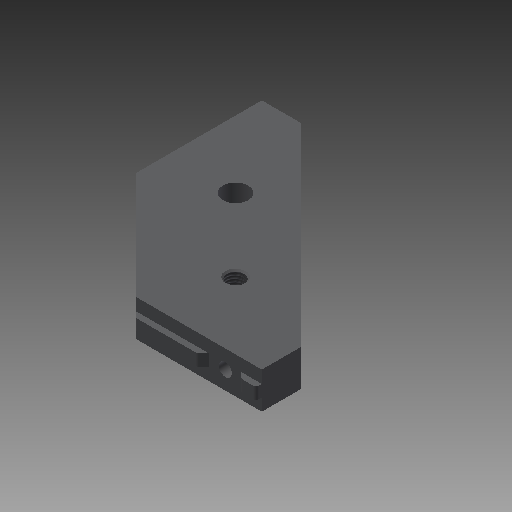
# Autodesk Inventor part: May Tec 1.47.225160.2_Floor mounting plate_schwarz-Pulverbeschichtet
Saved by Autodesk Inventor 2018 (Build 220112000, 112)
## iProperties
Category: PARTsolutions
Company: MAYTEC
Created: 2012-12-06
Part Number: May Tec 1.47.225160.2_Floor mounting plate_schwarz-Pulverbeschichtet
Catalog Web Link: www.cadenas.de
Description: Floor mounting plate-Floor mounting plate
Vendor: MAYTEC
Document SubType Name: Modeling
Designer: PARTuser1
Manufacturer: MAYTEC
Density: 1 g/cm^3
Material: Generic
Appearance: RGB(30.59999931603645,30.59999931603645,30.59999931603645)
PSOL_IDENT_0: {\\10.0.0.242\data_v9\23d-libs\maytec\maytec_3d\einbauzubehoer\platten\1.47.225.prj},292 {VTYP=3D},{
PSOL_IDENT_1: NB=May Tec 1.47.225160.2_Floor mounting plate_schwarz-Pulverbeschichtet},{LINA=May Tec 1.47.225160.2
PSOL_IDENT_2: _Floor mounting plate_schwarz-Pulverbeschichtet},{NN=Floor mounting plate},{DATE=14.09.2010 08:34:44
PSOL_IDENT_3: },{GEOMDATE=28.01.2010 00:00:00},{VERSION=},{LINEID=20},{LINESUBID=-1},{WBVAR=}  {NB=May Tec 1.47.22
PSOL_IDENT_4: 5160.2_Floor mounting plate_schwarz-Pulverbeschichtet},{LINA=May Tec 1.47.225160.2_Floor mounting pl
PSOL_IDENT_5: ate_schwarz-Pulverbeschichtet},{KT=DUMMY},{PARTNR=1.47.225160.2},{DESCRIPTION=Bodenbefestigungsplatt
PSOL_IDENT_6: e},{TYP=schwarz-Pulverbeschichtet},{COL=0.12,0.12,0.12,0.00},{XTRANS=Floor mounting plate}
CNS_NT: Floor mounting plate
CNS_NB: May Tec 1.47.225160.2_Floor mounting plate_schwarz-Pulverbeschichtet
CNS_NBSYN: May Tec $PARTNR._$XTRANS._$TYP.
CNS_LINA: May Tec 1.47.225160.2_Floor mounting plate_schwarz-Pulverbeschichtet
CNS_PARTNR: 1.47.225160.2
CNS_DESCRIPTION: Floor mounting plate
CNS_TYP: schwarz-Pulverbeschichtet
CNS_COL: 0.12,0.12,0.12,0.00
CNS_XTRANS: Floor mounting plate
SUPPLIER: MAYTEC
ARTICLENO: May Tec 1.47.225160.2_Floor mounting plate_schwarz-Pulverbeschichtet
BOMINFO: May Tec 1.47.225160.2_Floor mounting plate_schwarz-Pulverbeschichtet
CREATOR: CADENAS GmbH
Title: May Tec 1.47.225160.2_Floor mounting plate_schwarz-Pulverbeschichtet
Author: Cadenas PARTsolutions
Comments: Floor mounting plate
Autodesk Inventor part; units mm, degrees
sketch "Skizze_1" plane through (0, 0, 0) normal (0, 1, 0) x (-1, 0, 0)
  line L0 (73.8629, -73.8629) -> (0, 0)
  line L1 (0, 0) -> (-86.1371, 0)
  line L2 (-86.1371, 0) -> (-86.1371, -27)
  line L3 (-86.1371, -27) -> (46.8629, -160)
  line L4 (46.8629, -160) -> (73.8629, -160)
  line L5 (73.8629, -160) -> (73.8629, -73.8629)
  circle A0 centre (27.8629, -96) radius 8.7
  constraints: 12 end point, 1 centre point
extrude "Extrusion1" add sketch "Skizze_1" along normal mid plane 25
sketch "Skizze_2" plane through (0, 0, 0) normal (0, 1, 0) x (1, 0, 0)
  line L0 (72.1371, 0) -> (75.5513, -3.4142)
  arc A0 (75.5513, -3.4142) -> (76.9655, -4) centre (76.9655, -2) ccw
  line L1 (76.9655, -4) -> (84.1371, -4)
  arc A1 (84.1371, -4) -> (86.1371, -2) centre (84.1371, -2) ccw
  line L2 (86.1371, -2) -> (86.1371, 0)
  line L3 (86.1371, 0) -> (72.1371, 0)
  constraints: 8 end point, 4 point on circle, 2 centre point
extrude "Extrusion2" add sketch "Skizze_2" along normal mid plane 8
sketch "Skizze_3" plane through (0, 0, 0) normal (0, 1, 0) x (1, 0, 0)
  line L0 (0, 0) -> (3.4142, -3.4142)
  arc A0 (3.4142, -3.4142) -> (4.8284, -4) centre (4.8284, -2) ccw
  line L1 (4.8284, -4) -> (44.8087, -4)
  arc A1 (44.8087, -4) -> (46.2229, -3.4142) centre (44.8087, -2) ccw
  line L2 (46.2229, -3.4142) -> (49.6371, 0)
  line L3 (49.6371, 0) -> (0, 0)
  constraints: 8 end point, 4 point on circle, 2 centre point
extrude "Extrusion3" add sketch "Skizze_3" along normal mid plane 8
sketch "Skizze_4" plane through (0, 0, 0) normal (0, 1, 0) x (1, 0, 0)
  arc A0 (-77.8629, 150.8284) -> (-77.2771, 149.4142) centre (-75.8629, 150.8284) ccw
  line L0 (-77.2771, 149.4142) -> (-73.8629, 146)
  line L1 (-73.8629, 146) -> (-73.8629, 160)
  line L2 (-73.8629, 160) -> (-75.8629, 160)
  arc A1 (-75.8629, 160) -> (-77.8629, 158) centre (-75.8629, 158) ccw
  line L3 (-77.8629, 158) -> (-77.8629, 150.8284)
  constraints: 8 end point, 4 point on circle, 2 centre point
extrude "Extrusion4" add sketch "Skizze_4" along normal mid plane 8
sketch "Skizze_5" plane through (0, 0, 0) normal (0, 1, 0) x (1, 0, 0)
  line L0 (-77.8629, 118.6716) -> (-77.8629, 78.6913)
  arc A0 (-77.8629, 78.6913) -> (-77.2771, 77.2771) centre (-75.8629, 78.6913) ccw
  line L1 (-77.2771, 77.2771) -> (-73.8629, 73.8629)
  line L2 (-73.8629, 73.8629) -> (-73.8629, 123.5)
  line L3 (-73.8629, 123.5) -> (-77.2771, 120.0858)
  arc A1 (-77.2771, 120.0858) -> (-77.8629, 118.6716) centre (-75.8629, 118.6716) ccw
  constraints: 8 end point, 4 point on circle, 2 centre point
extrude "Extrusion5" add sketch "Skizze_5" along normal mid plane 8
sketch "Sketch6" plane through (0, -12.5, 0) normal (0, 0, 1) x (1, 0, 0)
  point P0 (61.1371, 12.5)
hole "Drilling 1" at (61.1371, 0, 0) direction (0, 0, -1) diameter 9 depth 92.3404
sketch "Skizze_7" plane through (0, 0, 0) normal (0, 1, 0) x (1, 0, 0)
  line L0 (50, 135) -> (-50, 135)
  line L1 (-73.8629, 135) -> (-73.8629, 139.5)
  line L2 (-73.8629, 139.5) -> (0, 139.5)
  line L3 (0, 139.5) -> (0, 135)
  line L4 (0, 135) -> (-73.8629, 135)
  constraints: 10 end point
revolve "Revolution1" cut sketch "Skizze_7" angle 360 about axis through (50, 0, -135) along (1, 0, 0)
sketch "Skizze_8" plane through (0, 0, 0) normal (0, 1, 0) x (1, 0, 0)
  line L0 (-46.1238, 53.1949) -> (-36.2244, 43.2954)
  line L1 (-36.2244, 43.2954) -> (0.0798, 76.9104)
  arc A0 (3.0475, 73.9428) -> (0.0798, 76.9104) centre (1.5066, 75.3695) ccw
  line L2 (3.0475, 73.9428) -> (-30.5675, 37.6386)
  line L3 (-30.5675, 37.6386) -> (-20.668, 27.7391)
  line L4 (-20.668, 27.7391) -> (12.566, 58.1447)
  line L5 (12.566, 58.1447) -> (42.9716, 70.1655)
  line L6 (42.9716, 70.1655) -> (-3.6974, 116.8345)
  line L7 (-3.6974, 116.8345) -> (-15.7183, 86.4289)
  line L8 (-15.7183, 86.4289) -> (-46.1238, 53.1949)
  constraints: 18 end point, 2 point on circle, 1 centre point
extrude "Extrusion6" cut sketch "Skizze_8" along normal mid plane 10
sketch "Sketch9" plane through (0, 12.5, 0) normal (0, 1, 0) x (1, 0, 0)
  point P0 (22.1, 46)
hole "Drilling 3" at (22.1, 12.5, -46) direction (0, -1, 0) diameter 11.835 depth 25 countersink diameter 14 countersink angle 90 thread size "M14x2" class "6H" standard "ISO Metric profile"
sketch "Skizze_10" plane through (0, 0, 0) normal (0, 1, 0) x (1, 0, 0)
  line L0 (-3.5355, 8.5355) -> (0, 5)
  line L1 (0, 5) -> (37.9741, 5)
  line L2 (37.9741, 5) -> (46.8927, 13.9185)
  line L3 (46.8927, 13.9185) -> (69.5201, 13.9185)
  line L4 (69.5201, 13.9185) -> (84.3693, 28.7678)
  line L5 (84.3693, 28.7678) -> (45.4465, 67.6906)
  line L6 (45.4465, 67.6906) -> (24.3701, 36.4411)
  line L7 (24.3701, 36.4411) -> (-3.5355, 8.5355)
  constraints: 16 end point
extrude "Extrusion7" cut sketch "Skizze_10" along normal mid plane 10
sketch "Skizze_11" plane through (0, 0, 0) normal (0, 1, 0) x (1, 0, 0)
  line L0 (-68.8629, 73.8629) -> (-65.3274, 70.3274)
  line L1 (-65.3274, 70.3274) -> (-39.1198, 102.7044)
  line L2 (-39.1198, 102.7044) -> (-6.1723, 119.3094)
  line L3 (-6.1723, 119.3094) -> (-45.0951, 158.2322)
  line L4 (-45.0951, 158.2322) -> (-59.9444, 143.383)
  line L5 (-59.9444, 143.383) -> (-59.9444, 120.7556)
  line L6 (-59.9444, 120.7556) -> (-68.8629, 111.837)
  line L7 (-68.8629, 111.837) -> (-68.8629, 73.8629)
  constraints: 16 end point
extrude "Extrusion8" cut sketch "Skizze_11" along normal mid plane 10
ref_plane "side_2a_XY" through (61.137, 0, 0) normal (0, 0, 1) x (1, 0, 0)
ref_plane "side_2a_YZ" through (61.137, 0, 0) normal (1, 0, 0) x (0, 1, 0)
ref_plane "side_2a_ZX" through (61.137, 0, 0) normal (0, 1, 0) x (0, 0, 1)
ref_plane "side_2b_XY" through (61.137, 0, -13.919) normal (0, 0, -1) x (1, 0, 0)
ref_plane "side_2b_YZ" through (61.137, 0, -13.919) normal (1, 0, 0) x (0, -1, 0)
ref_plane "side_2b_ZX" through (61.137, 0, -13.919) normal (0, -1, 0) x (0, 0, -1)
ref_plane "side_5a_XY" through (-73.863, 0, -135) normal (-1, 0, 0) x (0, 0, -1)
ref_plane "side_5a_YZ" through (-73.863, 0, -135) normal (0, 0, -1) x (0, -1, 0)
ref_plane "side_5a_ZX" through (-73.863, 0, -135) normal (0, -1, 0) x (-1, 0, 0)
ref_plane "side_5b_XY" through (-59.944, 0, -135) normal (1, 0, 0) x (0, 0, -1)
ref_plane "side_5b_YZ" through (-59.944, 0, -135) normal (0, 0, -1) x (0, 1, 0)
ref_plane "side_5b_ZX" through (-59.944, 0, -135) normal (0, 1, 0) x (1, 0, 0)
ref_plane "side_1a_XY" through (22.137, 12, -46) normal (0, 1, 0) x (1, 0, 0)
ref_plane "side_1a_YZ" through (22.137, 12, -46) normal (1, 0, 0) x (0, 0, -1)
ref_plane "side_1a_ZX" through (22.137, 12, -46) normal (0, 0, -1) x (0, 1, 0)
ref_plane "side_1b_XY" through (-27.863, 12, -96) normal (0, 1, 0) x (1, 0, 0)
ref_plane "side_1b_YZ" through (-27.863, 12, -96) normal (1, 0, 0) x (0, 0, -1)
ref_plane "side_1b_ZX" through (-27.863, 12, -96) normal (0, 0, -1) x (0, 1, 0)
ref_plane "side_6a_XY" through (22.137, -12, -46) normal (0, -1, 0) x (1, 0, 0)
ref_plane "side_6a_YZ" through (22.137, -12, -46) normal (1, 0, 0) x (0, 0, 1)
ref_plane "side_6a_ZX" through (22.137, -12, -46) normal (0, 0, 1) x (0, -1, 0)
ref_plane "side_6b_XY" through (-27.863, -12, -96) normal (0, -1, 0) x (1, 0, 0)
ref_plane "side_6b_YZ" through (-27.863, -12, -96) normal (1, 0, 0) x (0, 0, 1)
ref_plane "side_6b_ZX" through (-27.863, -12, -96) normal (0, 0, 1) x (0, -1, 0)
body "Solid1"
